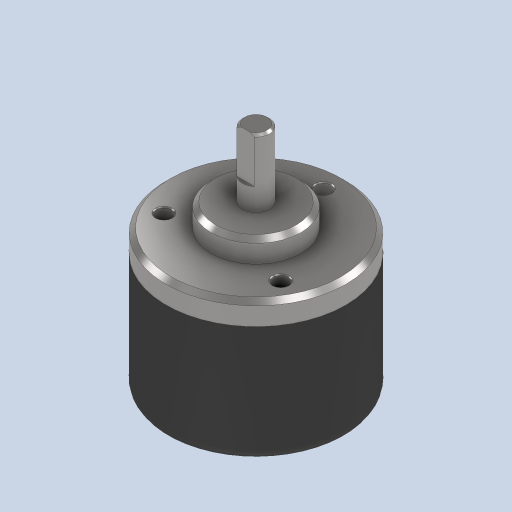
# Autodesk Inventor part: Encoder
Saved by Autodesk Inventor 2023 (Build 270158000, 158)
## iProperties
Created: 2024-02-17
Part Number: Encoder
Material: Stainless Steel
Document SubType Name: Modeling
Designer: Mateus Quintino
Density: 8 g/cm^3
Appearance: Semi-Polished
Author: Mateus Quintino
Autodesk Inventor part; units mm, degrees
ref_plane "YZ Plane" through (0, 0, 0) normal (1, 0, 0) x (0, 1, 0)
ref_plane "XZ Plane" through (0, 0, 0) normal (0, 1, 0) x (-1, 0, 0)
ref_plane "XY Plane" through (0, 0, 0) normal (0, 0, 1) x (1, 0, 0)
sketch "Sketch1" plane through (0, 0, 0) normal (0, 1, 0) x (-1, 0, 0)
  circle A0 centre (0, 0) radius 20
  dimension "d0" = 40
  constraints: 1 centre point, 1 coincident
  measures "d0" diameter of A0
extrude "Extrusion1" add sketch "Sketch1" along normal blind 26
sketch "Sketch2" plane through (0, 26, 0) normal (0, 1, 0) x (1, 0, 0)
  circle A0 centre (0, 0) radius 19.95
  dimension "d3" = 39.9
  constraints: 1 centre point, 1 coincident
  measures "d3" diameter of A0
extrude "Extrusion2" add sketch "Sketch2" along normal blind 5
sketch "Sketch3" plane through (0, 31, 0) normal (0, 1, 0) x (1, 0, 0)
  circle A0 centre (0, 0) radius 10
  dimension "d6" = 20
  constraints: 1 centre point, 1 coincident
  measures "d6" diameter of A0
extrude "Extrusion3" add sketch "Sketch3" along normal blind 5
sketch "Sketch4" plane through (0, 36, 0) normal (0, 1, 0) x (1, 0, 0)
  circle A0 centre (0, 0) radius 3
  dimension "d9" = 6
  constraints: 1 centre point, 1 coincident
  measures "d9" diameter of A0
extrude "Extrusion4" add sketch "Sketch4" along normal blind 15
sketch "Sketch5" plane through (0, 51, 0) normal (0, 1, 0) x (1, 0, 0)
  circle A0 centre (0, 0) radius 3 projected
  circle A1 centre (0, 0) radius 3 projected
  line L0 (-1.9261, -2.3) -> (1.9261, -2.3)
  dimension "d12" = 2.3
  constraints: 2 end point, 2 point on circle, 1 horizontal, 2 other
  measures "d12" distance from line of L0 point (0, 0)
extrude "Extrusion5" cut sketch "Sketch5" against normal blind 10 contours L0 A0 picked at (0.4482, -2.4273)
fillet "Fillet1" radius 2 1 edges at (20, 0, 0)
chamfer "Chamfer1" distance 1 angle 45 2 edges at (-19.95, 31, 0) (-10, 36, 0)
chamfer "Chamfer2" distance 0.5 angle 45 2 edges at (2.7183, 51, 1.2692) (-1.2692, 51, -2.7183)
sketch "Sketch6" plane through (0, 31, 0) normal (0, 1, 0) x (1, 0, 0)
  point P0 (0, 0)
  point P1 (0, 15)
  point P2 (-12.9904, -7.5)
  point P3 (12.9904, -7.5)
  dimension "d23" = 15
  dimension "d26" = 360
  constraints: 1 vertical alignment, 4 other
  measures "d23" distance of point (0, 0) point (0, 15)
hole "Hole1" at (0, 31, -15) at (-12.9904, 31, 7.5) at (12.9904, 31, 7.5) direction (0, -1, 0) diameter 3.4 depth 5 tip angle 118 countersink diameter 3.8 countersink angle 90 clearance for "Countersunk Raised Head Screw ISO 2010/7047" size "M3" standard "ISO"
body "Solid1"
